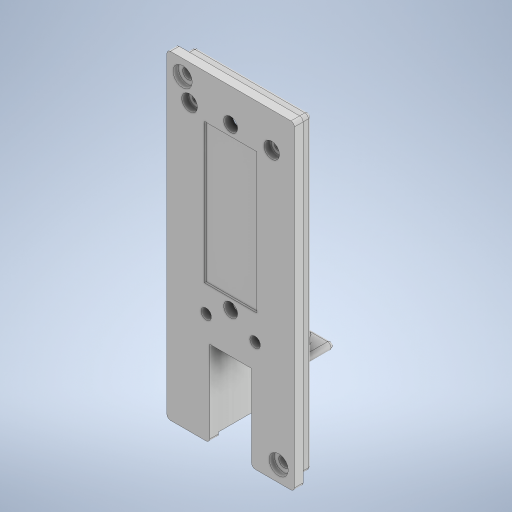
# Autodesk Inventor part: Base
Saved by Autodesk Inventor 2024 (Build 280153000, 153)
## iProperties
Created: 2024-01-29
Part Number: Base
Material: Generisch
Document SubType Name: Modeling
Designer: month
Density: 1 g/cm^3
Appearance: Vorgabe
Author: month
Autodesk Inventor part; units mm, degrees
ref_plane "YZ Plane" through (0, 0, 0) normal (1, 0, 0) x (0, 1, 0)
ref_plane "XZ Plane" through (0, 0, 0) normal (0, 1, 0) x (-1, 0, 0)
ref_plane "XY Plane" through (0, 0, 0) normal (0, 0, 1) x (1, 0, 0)
sketch "Skizze1" plane through (0, 0, 0) normal (0, 1, 0) x (-1, 0, 0)
  line L0 (0, 0) -> (36.5, 0)
  line L1 (36.5, 0) -> (36.5, 91.5)
  line L2 (36.5, 91.5) -> (0, 91.5)
  line L3 (0, 91.5) -> (0, 0)
  dimension "d0" = 91.5
  dimension "d1" = 36.5
  constraints: 8 end point, 2 parallel, 1 horizontal, 1 perpendicular
  measures "d0" distance of L0.end L1.end
  measures "d1" distance of L1.end L2.end
extrude "Extrusion1" add sketch "Skizze1" along normal blind 2.5
sketch "Skizze2" plane through (0, 2.5, 0) normal (0, 1, 0) x (1, 0, 0)
  line L0 (-35, -90) -> (-1.5, -90)
  line L1 (-1.5, -90) -> (-1.5, -1.5)
  line L2 (-1.5, -1.5) -> (-35, -1.5)
  line L3 (-35, -1.5) -> (-35, -90)
  line L4 (-36.5, -91.5) -> (0, -91.5) projected
  line L5 (0, 0) -> (-36.5, 0) projected
  line L6 (-36.5, 0) -> (-36.5, -91.5) projected
  line L7 (0, -91.5) -> (0, 0) projected
  dimension "d4" = 1.5
  dimension "d5" = 1.5
  dimension "d6" = 1.5
  dimension "d7" = 1.5
  constraints: 8 end point, 2 parallel, 1 horizontal, 1 perpendicular
  measures "d4" distance between parallel lines of L4 L0
  measures "d5" distance between parallel lines of L5 L2
  measures "d6" distance between parallel lines of L6 L3
  measures "d7" distance between parallel lines of L7 L1
extrude "Extrusion2" add sketch "Skizze2" along normal blind 4 contours L3 L2 L1 L0
sketch "Skizze3" plane through (0, 6.5, 0) normal (0, 1, 0) x (1, 0, 0)
  line L0 (-33.5, -88.5) -> (-3, -88.5)
  line L1 (-3, -88.5) -> (-3, -3)
  line L2 (-3, -3) -> (-33.5, -3)
  line L3 (-33.5, -3) -> (-33.5, -88.5)
  line L4 (-1.5, -1.5) -> (-35, -1.5) projected
  line L5 (-35, -1.5) -> (-35, -90) projected
  line L6 (-1.5, -90) -> (-1.5, -1.5) projected
  line L7 (-35, -90) -> (-1.5, -90) projected
  point P0 (0, 0)
  dimension "d10" = 1.5
  dimension "d11" = 1.5
  dimension "d12" = 1.5
  dimension "d13" = 1.5
  constraints: 8 end point, 2 parallel, 1 horizontal, 1 perpendicular
  measures "d10" distance between parallel lines of L4 L2
  measures "d11" distance between parallel lines of L5 L3
  measures "d12" distance between parallel lines of L6 L1
  measures "d13" distance between parallel lines of L7 L0
extrude "Extrusion3" cut sketch "Skizze3" against normal blind 4 contours L3 L2 L1 L0
sketch "Skizze7" plane through (0, 2.5, 0) normal (0, 1, 0) x (1, 0, 0)
  line L0 (-33.5, -88.5) -> (-33.5, -3) projected
  line L1 (-3, -3) -> (-3, -88.5) projected
  line L2 (-33.5, -26.5) -> (-3, -26.5)
  line L3 (-3, -26.5) -> (-3, -28.5)
  line L4 (-3, -28.5) -> (-33.5, -28.5)
  line L5 (-33.5, -28.5) -> (-33.5, -26.5)
  line L6 (-3, -88.5) -> (-33.5, -88.5) projected
  point P0 (0, 0)
  point P1 (-33.5, -28.5)
  point P2 (-3, -26.5)
  dimension "d29" = 60
  dimension "d30" = 2
  constraints: 8 end point, 2 parallel, 2 point on line, 1 horizontal, 1 perpendicular
  measures "d29" distance between parallel lines of L6 L4
  measures "d30" distance between parallel lines of L4 L2
extrude "Extrusion7" add sketch "Skizze7" along normal blind 12 contours L0 L2 L1 L4
sketch "Skizze9" plane through (-33.5, 2.5, 28.5) normal (0, 0, 1) x (1, 0, 0)
  line L0 (2.75, 6) -> (6.75, 6)
  line L1 (6.75, 6) -> (6.75, 4.5)
  line L2 (6.75, 4.5) -> (2.75, 4.5)
  line L3 (2.75, 4.5) -> (2.75, 6)
  line L4 (23.75, 6) -> (27.75, 6)
  line L5 (27.75, 6) -> (27.75, 4.5)
  line L6 (27.75, 4.5) -> (23.75, 4.5)
  line L7 (23.75, 4.5) -> (23.75, 6)
  line L8 (0, 12) -> (30.5, 12) projected
  line L9 (15.25, 12) -> (15.25, 0) construction
  line L10 (30.5, 0) -> (0, 0) projected
  point P0 (33.5, -2.5)
  point P1 (23.75, 5.25)
  point P2 (6.75, 5.25)
  dimension "d39" = 17
  dimension "d40" = 4
  dimension "d41" = 4
  dimension "d42" = 1.5
  dimension "d43" = 1.5
  dimension "d132" = 6
  constraints: 18 end point, 4 midpoint, 4 parallel, 2 horizontal, 2 perpendicular, 2 point on line, 1 symmetric about line
  measures "d39" distance of point (23.75, 5.25) point (6.75, 5.25)
  measures "d40" distance of L4.start L4.end
  measures "d41" distance of L0.start L0.end
  measures "d42" distance of L6.end L4.start
  measures "d43" distance of L0.end L1.end
  measures "d132" distance between parallel lines of L10 L0
extrude "Extrusion9" add sketch "Skizze9" along normal blind 2
sketch "Skizze11" plane through (0, 2.5, 0) normal (0, 1, 0) x (1, 0, 0)
  line L0 (-33.5, -26.5) -> (-3, -26.5) projected
  line L1 (-26.2, -26.5) -> (-10.3, -26.5)
  line L2 (-10.3, -26.5) -> (-10.3, -2.8679)
  line L3 (-10.3, -2.8679) -> (-26.2, -2.8679)
  line L4 (-26.2, -2.8679) -> (-26.2, -26.5)
  line L5 (-3, -88.5) -> (-33.5, -88.5) projected
  line L6 (-18.25, -88.5) -> (-18.25, -2.8679)
  line L7 (-33.5, -26.5) -> (-33.5, -3) projected
  point P0 (0, 0)
  point P1 (-36.5, 0)
  point P2 (-10.3, -26.5)
  dimension "d46" = 7.3
  constraints: 10 end point, 2 midpoint, 2 parallel, 2 perpendicular, 1 horizontal, 1 point on line, 1 other
  measures "d46" distance between parallel lines of L7 L4
extrude "Extrusion10" add sketch "Skizze11" along normal blind 12
sketch "Skizze12" plane through (-10.3, 6.5, 2.8679) normal (0, 0, -1) x (-1, 0, 0)
  line L0 (-7.3, 0) -> (23.2, 0) projected
  line L1 (0.6699, 0) -> (16.1486, 0)
  line L2 (23.2, 8) -> (-7.3, 8) projected
  line L3 (7.95, 8) -> (7.95, 0) construction
  line L4 (0.5, 0) -> (15.4, 0)
  line L5 (15.4, 0) -> (15.4, 7.5)
  line L6 (15.4, 7.5) -> (0.5, 7.5)
  line L7 (0.5, 7.5) -> (0.5, 0)
  line L8 (0, 0) -> (0, 8) projected
  point P0 (-10.3, -6.5)
  point P1 (0.5, 0)
  point P2 (15.4, 0)
  dimension "d49" = 0.5
  dimension "d50" = 0.5
  constraints: 12 end point, 3 point on line, 2 horizontal, 2 parallel, 2 perpendicular, 1 midpoint, 1 other
  measures "d49" distance between parallel lines of L8 L7
  measures "d50" distance between parallel lines of L2 L6
extrude "Extrusion11" add sketch "Skizze12" along normal blind 1.368
sketch "Skizze14" plane through (0, 0, 0) normal (0, 0, -1) x (-1, 0, 0)
  line L0 (0, 0) -> (36.5, 0) projected
  line L1 (18.25, 0) -> (18.25, 14.5) construction
  line L2 (10.3, 14.5) -> (26.2, 14.5) projected
  line L3 (24.25, 0) -> (12.25, 0)
  line L4 (12.25, 0) -> (12.25, 12)
  line L5 (12.25, 12) -> (24.25, 12)
  line L6 (24.25, 12) -> (24.25, 0)
  dimension "d53" = 12
  dimension "d54" = 12
  constraints: 10 end point, 2 midpoint, 2 parallel, 1 horizontal, 1 perpendicular, 1 point on line, 1 other
  measures "d53" distance between parallel lines of L4 L6
  measures "d54" distance between parallel lines of L0 L5
extrude "Extrusion12" cut sketch "Skizze14" against normal blind 24.5
sketch "Skizze15" plane through (0, 0, 24.5) normal (0, 0, -1) x (-1, 0, 0)
  line L0 (24.25, 0) -> (12.25, 0) projected
  line L1 (18.25, 0) -> (18.25, 12)
  line L2 (12.25, 12) -> (24.25, 12) projected
  line L3 (12.25, 12) -> (24.25, 12)
  line L4 (24.25, 12) -> (24.25, 2.5)
  line L5 (24.25, 2.5) -> (12.25, 2.5)
  line L6 (12.25, 2.5) -> (12.25, 12)
  point P0 (0, 0)
  dimension "d57" = 2.5
  constraints: 10 end point, 2 midpoint, 2 parallel, 1 horizontal, 1 perpendicular
  measures "d57" distance between parallel lines of L0 L5
extrude "Extrusion13" cut sketch "Skizze15" against normal blind 7.5
sketch "Skizze16" plane through (0, 0, 0) normal (0, -1, 0) x (1, 0, 0)
  line L0 (-36.5, 91.5) -> (0, 91.5) projected
  line L1 (-18.25, 91.5) -> (-18.25, 24.5)
  line L2 (-24.25, 24.5) -> (-12.25, 24.5) projected
  line L3 (-10.75, 79) -> (-25.75, 79)
  line L4 (-25.75, 79) -> (-25.75, 39)
  line L5 (-25.75, 39) -> (-10.75, 39)
  line L6 (-10.75, 39) -> (-10.75, 79)
  circle A0 centre (-18.25, 36.5) radius 2
  circle A1 centre (-18.25, 81.5) radius 2
  point P0 (0, 0)
  dimension "d60" = 15
  dimension "d61" = 40
  dimension "d62" = 12.5
  dimension "d72" = 2.5
  dimension "d73" = 4
  dimension "d74" = 2.5
  dimension "d75" = 4
  constraints: 10 end point, 2 centre point, 2 midpoint, 2 parallel, 2 point on line, 1 horizontal, 1 perpendicular, 1 other
  measures "d60" distance between parallel lines of L6 L4
  measures "d61" distance between parallel lines of L5 L3
  measures "d62" distance between parallel lines of L0 L3
  measures "d72" distance from line of A0.centre L5
  measures "d73" diameter of A0
  measures "d74" distance from line of L3 A1.centre
  measures "d75" diameter of A1
extrude "Extrusion14" cut sketch "Skizze16" against normal blind 0.5 contours L3 L6 L5 L1 | L1 L5 L4 L3
fillet "Rundung4" radius 1 6 edges at (-36.5, 1.25, 0) (-36.5, 1.25, 91.5) (0, 1.25, 91.5) (0, 1.25, 0) (-12.25, 1.25, 0) (-24.25, 1.25, 0)
fillet "Rundung5" radius 1 9 edges at (-35, 4.5, 1.5) (-1.5, 4.5, 1.5) (-35, 4.5, 90) (-30.35, 6.5, 1.5) (-35, 6.5, 45.75) (-6.15, 6.5, 1.5) (-1.5, 6.5, 45.75) (-1.5, 4.5, 90) (-18.25, 6.5, 90)
sketch "Skizze17" plane through (0, 0, 0) normal (0, -1, 0) x (1, 0, 0)
  line L0 (-24.25, 24.5) -> (-12.25, 24.5) projected
  line L1 (-18.25, 24.5) -> (-18.25, 91.5) construction
  line L2 (-35.5, 91.5) -> (-1, 91.5) projected
  circle A0 centre (-18.25, 82) radius 2
  circle A1 centre (-18.25, 36) radius 2
  line L3 (-25.75, 79) -> (-10.75, 79) projected
  line L4 (-10.75, 39) -> (-25.75, 39) projected
  point P0 (0, 0)
  dimension "d76" = 3
  dimension "d77" = 4
  dimension "d78" = 3
  dimension "d79" = 4
  constraints: 2 centre point, 2 end point, 2 midpoint, 2 point on line
  measures "d76" distance from line of A0.centre L3
  measures "d77" diameter of A0
  measures "d78" distance from line of A1.centre L4
  measures "d79" diameter of A1
extrude "Extrusion15" cut sketch "Skizze17" against normal blind 10
fillet "Rundung8" radius 1 9 edges at (-29.85, 14.5, 26.5) (-33.5, 14.5, 27.5) (-18.25, 14.5, 28.5) (-6.65, 14.5, 26.5) (-3, 14.5, 27.5) (-33.5, 10.5, 26.5) (-33.5, 10.5, 28.5) (-3, 10.5, 26.5) (-3, 10.5, 28.5)
sketch "Skizze18" plane through (0, 2.5, 0) normal (0, 1, 0) x (1, 0, 0)
  line L0 (-4.5, -2.9208) -> (-4.5, -26.5) construction
  line L1 (-10.3, -26.5) -> (-3, -26.5) projected
  line L2 (-3, -3) -> (-3, -26.5) projected
  circle A0 centre (-4.5, -4.5) radius 1.5
  line L3 (-10.3, -3) -> (-3, -3) projected
  point P0 (0, 0)
  dimension "d83" = 1.5
  dimension "d84" = 1.5
  dimension "d85" = 3
  constraints: 2 end point, 2 point on line, 1 centre point, 1 vertical
  measures "d83" distance between parallel lines of L2 L0
  measures "d84" distance from line of L3 A0.centre
  measures "d85" diameter of A0
extrude "Extrusion17" cut sketch "Skizze18" along normal mid plane 12 contours A0
sketch "Skizze19" plane through (0, 0, 0) normal (0, -1, 0) x (1, 0, 0)
  arc A0 (-4.5, 3) -> (-3, 4.5) centre (-4.5, 4.5) ccw
  circle A1 centre (-4.5, 4.5) radius 2.75
  circle A2 centre (-4.5, 4.5) radius 1.5 projected
  point P0 (0, 0)
  dimension "d90" = 5.5
  constraints: 2 centre point, 2 point on circle, 1 coincident, 1 concentric
  measures "d90" diameter of A1
extrude "Extrusion18" cut sketch "Skizze19" against normal blind 1.5 contours A2 A0 | A1
sketch "Skizze20" plane through (0, 2.5, 0) normal (0, 1, 0) x (1, 0, 0)
  circle A0 centre (-30, -81.5) radius 0.75 projected
  line L0 (-30, -81.5) -> (-33.5, -81.5) construction
  line L1 (-33.5, -88.5) -> (-33.5, -28.5) projected
  circle A1 centre (-30, -81.5) radius 1.5 projected
  line L2 (-30, -81.5) -> (-30, -88.5) construction
  line L3 (-3, -88.5) -> (-33.5, -88.5) projected
  circle A2 centre (-32, -87) radius 1.5
  point P0 (0, 0)
  dimension "d93" = 1.5
  dimension "d94" = 1.5
  dimension "d95" = 3
  constraints: 4 end point, 2 point on line, 1 centre point, 1 horizontal, 1 vertical
  measures "d93" distance from line of A2.centre L3
  measures "d94" distance from line of L1 A2.centre
  measures "d95" diameter of A2
extrude "Extrusion19" cut sketch "Skizze20" against normal blind 2 contours A2
sketch "Skizze21" plane through (0, 0, 0) normal (0, -1, 0) x (1, 0, 0)
  arc A0 (-33.5, 87) -> (-32, 88.5) centre (-32, 87) ccw projected
  circle A1 centre (-32, 87) radius 2.75
  point P0 (0, 0)
  dimension "d98" = 5.5
  constraints: 1 centre point, 1 coincident
  measures "d98" diameter of A1
extrude "Extrusion20" cut sketch "Skizze21" against normal blind 1.5
sketch "Skizze22" plane through (0, 2.5, 0) normal (0, 1, 0) x (1, 0, 0)
  line L0 (-10.3, -3) -> (-3, -3) projected
  line L1 (-7, -3) -> (-7, -7)
  line L2 (-7, -7) -> (-3, -7)
  line L3 (-3, -3) -> (-3, -26.5) projected
  line L4 (-3, -3) -> (-3, -7)
  line L5 (-3, -3) -> (-7, -3)
  point P0 (0, 0)
  dimension "d101" = 4
  dimension "d102" = 4
  constraints: 8 end point, 3 perpendicular, 2 point on line, 1 vertical
  measures "d101" distance of L1.start L1.end
  measures "d102" distance of L1.end L2.end
extrude "Extrusion21" add sketch "Skizze22" along normal blind 4
sketch "Skizze23" plane through (-4.5, 2.5, 4.5) normal (0, -1, 0) x (1, 0, 0)
  circle A0 centre (0, 0) radius 1.5
  circle A1 centre (0, 0) radius 1.5 projected
  line L0 (0, 1.5) -> (0, -1.5) construction
  line L1 (-1.5, 0) -> (1.5, 0) construction
  point P0 (4.5, -4.5)
  dimension "d105" = 3
  constraints: 4 end point, 4 point on circle, 3 midpoint, 1 centre point, 1 coincident, 1 horizontal, 1 vertical
  measures "d105" diameter of A0
extrude "Extrusion22" cut sketch "Skizze23" against normal blind 12
fillet "Rundung9" radius 2 1 edges at (-7, 4.5, 7)
sketch "Skizze24" plane through (0, 2.5, 0) normal (0, 1, 0) x (1, 0, 0)
  line L0 (-33.5, -88.5) -> (-33.5, -28.5) projected
  line L1 (-33.5, -84.5) -> (-29.5, -84.5)
  line L2 (-29.5, -84.5) -> (-29.5, -88.5)
  line L3 (-3, -88.5) -> (-33.5, -88.5) projected
  line L4 (-29.5, -88.5) -> (-33.5, -88.5)
  line L5 (-33.5, -88.5) -> (-33.5, -84.5)
  point P0 (0, 0)
  dimension "d109" = 4
  dimension "d110" = 4
  constraints: 8 end point, 2 horizontal, 2 perpendicular, 2 point on line
  measures "d109" distance of L1.start L1.end
  measures "d110" distance of L1.end L2.end
extrude "Extrusion23" add sketch "Skizze24" along normal blind 4
sketch "Skizze25" plane through (-32, 2.5, 87) normal (0, -1, 0) x (1, 0, 0)
  circle A0 centre (0, 0) radius 1.5 projected
  line L0 (0, 1.5) -> (0, -1.5) construction
  line L1 (-1.5, 0) -> (1.5, 0) construction
  circle A1 centre (0, 0) radius 1.5
  point P0 (32, -87)
  dimension "d113" = 3
  constraints: 4 end point, 4 point on circle, 3 midpoint, 1 centre point, 1 coincident, 1 horizontal, 1 vertical
  measures "d113" diameter of A1
extrude "Extrusion24" cut sketch "Skizze25" against normal blind 10
fillet "Rundung10" radius 2 1 edges at (-29.5, 4.5, 84.5)
sketch "Skizze26" plane through (0, 2.5, 0) normal (0, 1, 0) x (1, 0, 0)
  line L0 (-3, -88.5) -> (-29.5, -88.5) projected
  line L1 (-30, -88.5) -> (-30, -81.5)
  line L2 (-30, -81.5) -> (-33.5, -81.5)
  line L3 (-33.5, -84.5) -> (-33.5, -28.5) projected
  circle A0 centre (-30, -81.5) radius 1.25
  line L4 (-6.5, -88.5) -> (-6.5, -81.5)
  line L5 (-6.5, -81.5) -> (-3, -81.5)
  line L6 (-3, -28.5) -> (-3, -88.5) projected
  circle A1 centre (-6.5, -81.5) radius 1.25
  point P0 (0, 0)
  dimension "d117" = 7
  dimension "d118" = 3.5
  dimension "d119" = 2.5
  dimension "d122" = 7
  dimension "d123" = 3.5
  dimension "d124" = 2.5
  constraints: 8 end point, 4 point on line, 2 centre point, 2 coincident, 2 perpendicular, 2 vertical
  measures "d117" distance of L1.start L1.end
  measures "d118" distance of L1.end L2.end
  measures "d119" diameter of A0
  measures "d122" distance of L4.start L4.end
  measures "d123" distance of L4.end L5.end
  measures "d124" diameter of A1
extrude "Extrusion26" cut sketch "Skizze26" against normal blind 6 contours A1 L5 L4 | L4 L5 A1 | A0 L2 L1 | L1 L2 A0
sketch "Skizze27" plane through (0, 0, 0) normal (0, -1, 0) x (1, 0, 0)
  circle A0 centre (-6.5, 81.5) radius 1.25 projected
  circle A1 centre (-6.5, 81.5) radius 2.25
  circle A2 centre (-30, 81.5) radius 1.25 projected
  circle A3 centre (-30, 81.5) radius 2.25
  point P0 (0, 0)
  dimension "d127" = 4.5
  dimension "d128" = 4.5
  constraints: 2 centre point, 2 coincident
  measures "d127" diameter of A1
  measures "d128" diameter of A3
extrude "Extrusion27" cut sketch "Skizze27" against normal blind 2
fillet "Rundung12" radius 2 4 edges at (-30.75, 7, 29.5) (-26.75, 7, 29.5) (-9.75, 7, 29.5) (-5.75, 7, 29.5)
sketch "Skizze28" plane through (-33.5, 2.5, 28.5) normal (0, 0, 1) x (1, 0, 0)
  line L0 (2.75, 6) -> (6.75, 6) projected
  line L1 (4.75, 6) -> (4.75, 11) construction
  line L2 (7.3, 11) -> (1, 11) projected
  line L3 (23.75, 6) -> (27.75, 6) projected
  line L4 (25.75, 6) -> (25.75, 11) construction
  line L5 (29.5, 11) -> (23.2, 11) projected
  line L6 (2.75, 7.65) -> (6.75, 7.65)
  line L7 (6.75, 7.65) -> (6.75, 9.15)
  line L8 (6.75, 9.15) -> (2.75, 9.15)
  line L9 (2.75, 9.15) -> (2.75, 7.65)
  line L10 (23.75, 7.65) -> (27.75, 7.65)
  line L11 (27.75, 7.65) -> (27.75, 9.15)
  line L12 (27.75, 9.15) -> (23.75, 9.15)
  line L13 (23.75, 9.15) -> (23.75, 7.65)
  point P0 (33.5, -2.5)
  dimension "d134" = 1.65
  dimension "d135" = 1.65
  dimension "d136" = 1.5
  dimension "d137" = 1.5
  dimension "d138" = 4
  dimension "d139" = 4
  constraints: 20 end point, 5 parallel, 2 horizontal, 2 midpoint, 2 perpendicular, 2 point on line, 1 vertical, 2 other
  measures "d134" distance between parallel lines of L6 L0
  measures "d135" distance between parallel lines of L3 L10
  measures "d136" distance between parallel lines of L6 L8
  measures "d137" distance between parallel lines of L10 L12
  measures "d138" distance of L7.end L8.end
  measures "d139" distance of L11.end L12.end
extrude "Extrusion28" add sketch "Skizze28" along normal blind 2
fillet "Rundung13" radius 2 4 edges at (-26.75, 11.65, 29.5) (-5.75, 11.65, 29.5) (-9.75, 11.65, 29.5) (-30.75, 11.65, 29.5)
sketch "Skizze29" plane through (0, 2.5, 0) normal (0, 1, 0) x (1, 0, 0)
  circle A0 centre (-18.25, -36) radius 2 projected
  line L0 (-18.25, -36) -> (-18.25, -28.5) construction
  line L1 (-24.25, -28.5) -> (-12.25, -28.5) projected
  line L2 (-33.5, -84.5) -> (-33.5, -28.5) projected
  line L3 (-33.5, -31.5) -> (-3.1269, -31.5) construction
  line L4 (-24.25, -28.5) -> (-33.5, -28.5) projected
  circle A1 centre (-25.25, -31.5) radius 1.5
  circle A2 centre (-11.25, -31.5) radius 1.5
  point P0 (0, 0)
  dimension "d143" = 3
  dimension "d144" = 7
  dimension "d145" = 7
  dimension "d146" = 3
  dimension "d147" = 3
  constraints: 4 end point, 3 point on line, 2 centre point, 1 horizontal, 1 midpoint
  measures "d143" distance between parallel lines of L3 L4
  measures "d144" distance from line of L0 A1.centre
  measures "d145" distance from line of L0 A2.centre
  measures "d146" diameter of A1
  measures "d147" diameter of A2
extrude "Extrusion29" cut sketch "Skizze29" against normal blind 10 contours A1 | A2
